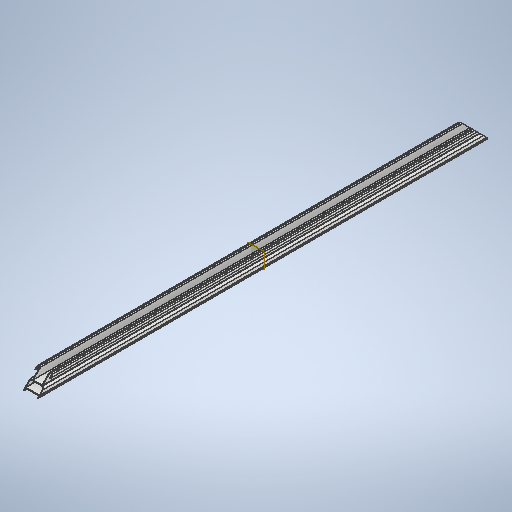
# Autodesk Inventor part: SP40-09 MARCO CORREDERA 1400 MM
Saved by Autodesk Inventor 2025 (Build 290162000, 162)
## iProperties
Created: 2026-01-17
Part Number: SP40-09 MARCO CORREDERA 1400 MM
Material: Aluminio
Document SubType Name: Modeling
Designer: ROLANDO
Density: 2.7 g/cm^3
Appearance: Satinado
Author: ROLANDO
Autodesk Inventor part; units mm, degrees
ref_plane "YZ Plane" through (0, 0, 0) normal (1, 0, 0) x (0, 1, 0)
ref_plane "XZ Plane" through (0, 0, 0) normal (0, 1, 0) x (-1, 0, 0)
ref_plane "XY Plane" through (0, 0, 0) normal (0, 0, 1) x (1, 0, 0)
sketch "Boceto1" plane through (0, 0, 0) normal (0, 0, 1) x (1, 0, 0)
  line L0 (-46, -14.91) -> (-46, -35.91)
  line L1 (-44.1, -31.91) -> (-2.9, -31.91)
  line L2 (-1, -35.91) -> (-1, -20.31)
  line L3 (-8.1, 6.6131) -> (-8.1, -14.91)
  line L4 (-44.6, -16.31) -> (-6.4, -16.31)
  line L5 (-2.4, -20.31) -> (-2.4, -30.01)
  line L6 (-2.9, -30.51) -> (-44.1, -30.51)
  line L7 (-44.6, -30.01) -> (-44.6, -16.31)
  arc A0 (-2.4, -20.31) -> (-6.4, -16.31) centre (-6.4, -20.31) ccw
  line L8 (-2.4, -32.41) -> (-2.4, -34.1632)
  line L9 (-3.5, -35.91) -> (-1, -35.91)
  line L10 (-9.5, -14.91) -> (-9.5, 7.7994)
  line L11 (-44.6, -32.41) -> (-44.6, -34.2323)
  line L12 (-43.5, -35.91) -> (-46, -35.91)
  line L13 (-43.5, -35.91) -> (-43.5, -35.4546)
  line L14 (-3.5, -35.91) -> (-3.5, -35.21)
  line L15 (-43.7447, -35.0247) -> (-44.3553, -34.6622)
  line L16 (-3.5, -35.21) -> (-2.6082, -34.5692)
  arc A1 (-2.9, -30.51) -> (-2.4, -30.01) centre (-2.9, -30.01) ccw
  arc A2 (-2.4, -32.41) -> (-2.9, -31.91) centre (-2.9, -32.41) ccw
  arc A3 (-2.6082, -34.5692) -> (-2.4, -34.1632) centre (-2.9, -34.1632) ccw
  arc A4 (-44.6, -30.01) -> (-44.1, -30.51) centre (-44.1, -30.01) ccw
  arc A5 (-44.1, -31.91) -> (-44.6, -32.41) centre (-44.1, -32.41) ccw
  arc A6 (-44.6, -34.2323) -> (-44.3553, -34.6622) centre (-44.1, -34.2323) ccw
  arc A7 (-43.5, -35.4546) -> (-43.7447, -35.0247) centre (-44, -35.4546) ccw
  line L17 (-9.5, 7.7994) -> (-4.75, 8.59)
  line L18 (-4.75, 8.59) -> (0, 7.7994)
  line L19 (-8.1, 6.6131) -> (-4.75, 7.1707)
  line L20 (-4.75, 7.1707) -> (-1.4, 6.6131)
  line L21 (0, 7.7994) -> (0, 0)
  line L22 (0, 0) -> (-1.4, 0)
  line L23 (-1.4, 0) -> (-1.4, 6.6131)
  line L24 (-8.1, -14.91) -> (-6.4, -14.91)
  arc A8 (-1, -20.31) -> (-6.4, -14.91) centre (-6.4, -20.31) ccw
  line L25 (-4.75, 16.5254) -> (-4.75, 0) construction
  line L26 (-38.9, 6.6131) -> (-38.9, -14.91)
  line L27 (-37.5, -14.91) -> (-37.5, 7.7994)
  line L28 (-37.5, 7.7994) -> (-42.25, 8.59)
  line L29 (-42.25, 8.59) -> (-47, 7.7994)
  line L30 (-38.9, 6.6131) -> (-42.25, 7.1707)
  line L31 (-42.25, 7.1707) -> (-45.6, 6.6131)
  line L32 (-47, 7.7994) -> (-47, 0)
  line L33 (-47, 0) -> (-45.6, 0)
  line L34 (-45.6, 0) -> (-45.6, 6.6131)
  line L35 (-42.25, 16.5254) -> (-42.25, 0) construction
  line L36 (-9.5, -14.91) -> (-37.5, -14.91)
  line L37 (-38.9, -14.91) -> (-46, -14.91)
  line L38 (-23.5, 14.1873) -> (-23.5, -36.7854) construction
  point P0 (-44.6, -34.5169)
  point P1 (-43.5, -35.17)
  dimension "d17" = 4
  dimension "d24" = 1.4
  dimension "d50" = 0.7
  dimension "d61" = 0.74
  dimension "d62" = 30.7
  dimension "d63" = 35.7
  dimension "d206" = 1.4
  dimension "d207" = 1.4
  dimension "d210" = 1.4
  dimension "d211" = 1.4
  dimension "d213" = 14.2
  dimension "d214" = 1.4
  dimension "d215" = 1.4
  dimension "d216" = 1.4
  dimension "d217" = 1.4
  dimension "d218" = 45
  dimension "d223" = 5.4
  dimension "d224" = 1.4
  dimension "d225" = 9.5
  dimension "d226" = 4.75
  dimension "d227" = 3.35
  dimension "d228" = 6.7
  dimension "d229" = 44.5
  dimension "d230" = 3.35
  dimension "d231" = 2.5
  dimension "d232" = 2.5
  dimension "d240" = 8.59
  dimension "d241" = 3.35
  dimension "d242" = 99.45
  dimension "d243" = 161.1
  dimension "d246" = 1.4
  dimension "d247" = 1.4
  dimension "d248" = 1.4
  dimension "d253" = 1.4
  dimension "d254" = 1.4
  dimension "d255" = 1.4
  dimension "d256" = 1.4
  dimension "d257" = 8.59
  dimension "d258" = 161.1
  dimension "d259" = 99.45
  dimension "d260" = 22.5
  dimension "d266" = 23.5
  dimension "d267" = 47
  dimension "d268" = 3.35
  dimension "d269" = 9.5
  dimension "d270" = 4.75
  dimension "d271" = 3.35
  dimension "d272" = 6.7
  dimension "d273" = 28
  dimension "d274" = 37.5
  dimension "d275" = 8.5
  dimension "d276" = 8.5
  dimension "d277" = 44.5
  dimension "d278" = 0.5
  dimension "d279" = 14.91
  dimension "d280" = 14.91
  dimension "d283" = 16.5254
  dimension "d284" = 0
  dimension "d285" = 14.1873
  dimension "d286" = 36.7854
  dimension "d287" = 16.5254
  dimension "d288" = 0
  constraints: 78 end point, 18 point on circle, 18 tangent, 10 parallel, 9 centre point, 6 equal radius, 6 point on line, 5 collinear, 5 perpendicular, 4 horizontal, 2 vertical, 1 coincident
  measures "d17" radius of A0
  measures "d24" distance between parallel lines of L1 L6
  measures "d50" distance of L9.start L14.end
  measures "d61" distance of L12.start point (-43.5, -35.17)
  measures "d62" angle of L12 L15
  measures "d63" angle of L9 L16
  measures "d206" distance between parallel lines of L21 L23
  measures "d207" distance between parallel lines of L3 L10
  measures "d210" distance between parallel lines of L17 L19
  measures "d211" distance between parallel lines of L18 L20
  measures "d213" distance between parallel lines of L4 L6
  measures "d214" distance between parallel lines of L8 L2
  measures "d215" distance between parallel lines of L2 L5
  measures "d216" distance between parallel lines of L0 L7
  measures "d217" distance between parallel lines of L0 L11
  measures "d218" distance between parallel lines of L2 L0
  measures "d223" radius of A8
  measures "d224" radial gap between concentric circles of A8 A0
  measures "d225" distance between parallel lines of L21 L10
  measures "d226" distance from line of L10 L17.end
  measures "d227" distance from line of L3 L19.end
  measures "d228" distance between parallel lines of L23 L3
  measures "d229" distance from line of L9 L17.end
  measures "d230" horizontal distance of L19.end L20.end
  measures "d231" distance of L9.start L2.start
  measures "d232" distance of L12.start L0.end
  measures "d240" distance from line of L17.end L22
  measures "d241" distance between parallel lines of L3 L25
  measures "d242" angle of L25 L18
  measures "d243" angle of L17 L18
  measures "d246" distance between parallel lines of L4 L37
  measures "d247" distance between parallel lines of L4 L36
  measures "d248" distance between parallel lines of L4 L24
  measures "d253" distance between parallel lines of L26 L27
  measures "d254" distance between parallel lines of L28 L30
  measures "d255" distance between parallel lines of L29 L31
  measures "d256" distance between parallel lines of L32 L34
  measures "d257" distance from line of L28.end L33
  measures "d258" angle of L29 L28
  measures "d259" angle of L35 L29
  measures "d260" distance between parallel lines of L2 L38
  measures "d266" distance between parallel lines of L38 L21
  measures "d267" distance between parallel lines of L21 L32
  measures "d268" distance between parallel lines of L26 L35
  measures "d269" distance between parallel lines of L32 L27
  measures "d270" distance between parallel lines of L35 L27
  measures "d271" distance between parallel lines of L34 L35
  measures "d272" distance between parallel lines of L26 L34
  measures "d273" distance between parallel lines of L10 L27
  measures "d274" distance between parallel lines of L25 L35
  measures "d275" distance between parallel lines of L0 L27
  measures "d276" distance between parallel lines of L2 L10
  measures "d277" distance from line of L12 L28.end
  measures "d278" radius of A1
  measures "d279" distance between parallel lines of L36 L22
  measures "d280" distance between parallel lines of L37 L22
  measures "d283" distance from line of L25.start L22
  measures "d284" distance from line of L25.end L22
  measures "d285" distance from line of L38.start L22
  measures "d286" distance from line of L38.end L22
  measures "d287" distance from line of L35.start L22
  measures "d288" distance from line of L35.end L22
extrude "Extrusión1" add sketch "Boceto1" against normal blind 1400
ref_plane "Plano de trabajo1" through (0, 0, -700) normal (0, 0, -1) x (-1, 0, 0)
sketch "Boceto2" plane through (0, 0, 0) normal (1, 0, 0) x (0, 1, 0)
  line L0 (-35.91, 0) -> (-20.31, 0) projected
  line L1 (-35.91, 0) -> (-35.91, -1400) projected
  line L2 (-20.31, -1400) -> (-35.91, -1400) projected
  line L3 (-20.31, 0) -> (-20.31, -1400) projected
  line L4 (-20.31, 0) -> (-14.91, 0) projected
  line L5 (-20.31, 0) -> (-20.31, -1400) projected
  line L6 (-14.91, -1400) -> (-20.31, -1400) projected
  line L7 (-14.91, 0) -> (-14.91, -1400) projected
  line L8 (-14.91, 0) -> (6.6131, 0) projected
  line L9 (-14.91, 0) -> (-14.91, -1400) projected
  line L10 (6.6131, -1400) -> (-14.91, -1400) projected
  line L11 (6.6131, 0) -> (6.6131, -1400) projected
  line L12 (0, 0) -> (7.7994, 0) projected
  line L13 (0, 0) -> (0, -1400) projected
  line L14 (7.7994, -1400) -> (0, -1400) projected
  line L15 (7.7994, 0) -> (7.7994, -1400) projected
  line L16 (7.7994, 0) -> (8.59, 0) projected
  line L17 (7.7994, 0) -> (7.7994, -1400) projected
  line L18 (8.59, -1400) -> (7.7994, -1400) projected
  line L19 (8.59, 0) -> (8.59, -1400) projected
  line L20 (-35.91, 0) -> (8.59, -44.5)
  line L21 (8.59, 0) -> (8.59, -44.5)
  line L22 (8.59, 0) -> (-35.91, 0)
  dimension "d291" = 45
  constraints: 6 end point, 1 perpendicular, 1 point on line
  measures "d291" angle of L0 L20
extrude "Extrusión2" cut sketch "Boceto2" against normal through all contours L0 L3 L20 | L4 L7 L20 L3 | L8 L13 L20 L7 | L8 L11 L20 L13 | L12 L15 L20 L11 | L16 L19 L20 L15
mirror "Simetría1" about plane through (0, 0, -700) normal (0, 0, -1) of "Extrusión2"
